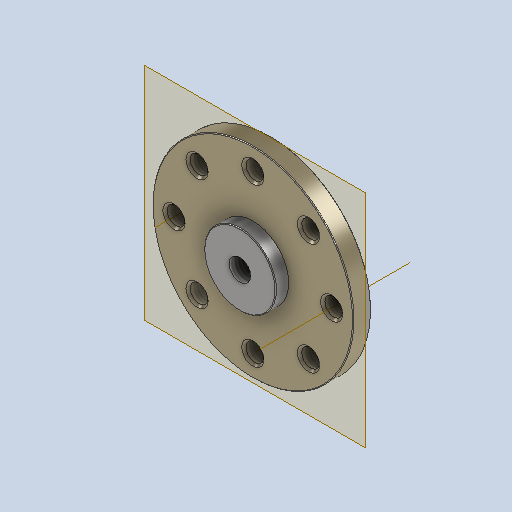
# Autodesk Inventor part: 64-106Horn
Saved by Autodesk Inventor 2024.3 (Build 283343000, 343)
## iProperties
Created: 2024-02-15
Part Number: 64-106Horn
Material: 강철, 합금
Document SubType Name: Modeling
Designer: ASUS
Appearance: 반연마
Surface Area: 15.9388 cm^2
Volume: 1.54868 cm^3
Author: ASUS
Autodesk Inventor part; units mm, degrees
ref_plane "YZ Plane" through (0, 0, 0) normal (1, 0, 0) x (0, 1, 0)
ref_plane "XZ Plane" through (0, 0, 0) normal (0, 1, 0) x (-1, 0, 0)
ref_plane "XY Plane" through (0, 0, 0) normal (0, 0, 1) x (1, 0, 0)
ref_plane "작업 평면1" through (0, 0, 0) normal (0, 0, 1) x (1, 0, 0)
sketch "스케치1" plane through (0, 0, 0) normal (0, 0, 1) x (1, 0, 0)
  circle A0 centre (-11, 0) radius 1.25 projected
  circle A1 centre (11, 0) radius 1.25 projected
  circle A2 centre (7.7782, -7.7782) radius 1.25 projected
  circle A3 centre (-7.7782, 7.7782) radius 1.25 projected
  circle A4 centre (-7.7782, -7.7782) radius 1.25 projected
  circle A5 centre (7.7782, 7.7782) radius 1.25 projected
  circle A6 centre (0, -11) radius 1.25 projected
  circle A7 centre (0, 11) radius 1.25 projected
  circle A8 centre (0, 0) radius 14 projected
  circle A9 centre (0, 0) radius 5 projected
ref_plane "작업 평면2" through (-14, -14, -2.5) normal (0, 0, -1) x (0, 1, 0)
extrude "돌출1" add sketch "스케치1" against normal up to surface (2.5 mm away) contours A8 | A9
sketch "스케치2" plane through (0, 0, 0) normal (0, 0, 1) x (1, 0, 0)
  circle A0 centre (0, 0) radius 5 projected
  circle A1 centre (0, 0) radius 2.75 projected
  circle A2 centre (0, 0) radius 1.5
  dimension "d2" = 3
  constraints: 1 centre point, 1 coincident
  measures "d2" diameter of A2
ref_plane "작업 평면3" through (-5, -5, 1.8) normal (0, 0, 1) x (1, 0, 0)
extrude "돌출2" add sketch "스케치2" along normal up to surface (1.8 mm away) contours A0 | A1
sketch "스케치3" plane through (0, 0, 1.8) normal (0, 0, 1) x (1, 0, 0)
  circle A0 centre (0, 0) radius 1.5 projected
  circle A1 centre (0, 0) radius 5 projected
  point P0 (0, 0)
extrude "돌출3" cut sketch "스케치3" against normal through all contours A0
thread "스레드1" size "M3x0.5" class "6H" standard "ANSI Metric M Profile" full length
fillet "모깎기1" radius 0.1 2 edges at (-14, 0, 0) (-14, 0, -2.5)
fillet "모깎기2" radius 0.1 1 edges at (-5, 0, 1.8)
thread "스레드2" size "M2.5x0.45" class "6H" standard "ANSI Metric M Profile" full length
thread "스레드3" size "M2.5x0.45" class "6H" standard "ANSI Metric M Profile" full length
thread "스레드4" size "M2.5x0.45" class "6H" standard "ANSI Metric M Profile" full length
thread "스레드5" size "M2.5x0.45" class "6H" standard "ANSI Metric M Profile" full length
thread "스레드6" size "M2.5x0.45" class "6H" standard "ANSI Metric M Profile" full length
thread "스레드7" size "M2.5x0.45" class "6H" standard "ANSI Metric M Profile" full length
thread "스레드8" size "M2.5x0.45" class "6H" standard "ANSI Metric M Profile" full length
thread "스레드9" size "M2.5x0.45" class "6H" standard "ANSI Metric M Profile" full length
chamfer "모따기1" distance 0.3 angle 45 8 edges at (-9.0282, 7.7782, 0) (-1.25, 11, 0) (6.5282, 7.7782, 0) (9.75, 0, 0) (6.5282, -7.7782, 0) (-1.25, -11, 0) (-9.0282, -7.7782, 0) (-12.25, 0, 0)
